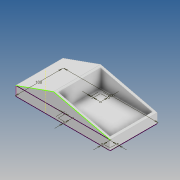
# Autodesk Inventor part: Cybertruck 1
Saved by Autodesk Inventor 2020 (Build 240168000, 168)
## iProperties
Created: 2019-11-26
Part Number: Cybertruck 1
Material: Generic
Document SubType Name: Modeling
Designer: Berkant
Density: 1 g/cm^3
Appearance: Default
Author: Berkant
Autodesk Inventor part; units mm, degrees
ref_plane "YZ Plane" through (0, 0, 0) normal (1, 0, 0) x (0, 1, 0)
ref_plane "XZ Plane" through (0, 0, 0) normal (0, 1, 0) x (-1, 0, 0)
ref_plane "XY Plane" through (0, 0, 0) normal (0, 0, 1) x (1, 0, 0)
sketch "Sketch1" plane through (0, 0, 0) normal (0, 1, 0) x (-1, 0, 0)
  line L0 (0, 0) -> (200, 0)
  line L1 (200, 0) -> (200, -100)
  line L2 (200, -100) -> (0, -100)
  line L3 (0, -100) -> (0, 0)
  dimension "d0" = 200
  dimension "d1" = 100
  constraints: 8 end point, 2 parallel, 1 horizontal, 1 perpendicular
  measures "d0" distance of L1.end L2.end
  measures "d1" distance of L0.end L1.end
extrude "Extrusion1" add sketch "Sketch1" along normal blind 20
sketch "Sketch2" plane through (-200, 0, 0) normal (0, 0, 1) x (1, 0, 0)
  line L0 (0, 0) -> (0, 20) projected
  line L1 (0, 0) -> (32, 0)
  line L2 (32, 0) -> (64, 0)
  line L3 (200, 0) -> (0, 0) projected
  line L4 (64, 0) -> (96, 0)
  line L5 (96, 0) -> (128, 0)
  line L6 (128, 0) -> (200, 0)
  line L7 (64, 0) -> (64, 80.3945) construction
  line L8 (200, 20) -> (0, 20) projected
  line L9 (0, 20) -> (200, 20)
  line L10 (0, 20) -> (200, 20) projected
  line L11 (0, 20) -> (200, 20)
  line L12 (0, 20) -> (80, 48.5382)
  line L13 (80, 48.5382) -> (200, 20)
  constraints: 20 end point, 3 collinear, 3 point on line, 1 horizontal, 1 vertical
extrude "Extrusion2" add sketch "Sketch2" against normal blind 100
sketch "Sketch4" plane through (0, 0, 0) normal (0, -1, 0) x (1, 0, 0)
  line L0 (0, 0) -> (-5, 0)
  line L1 (-5, 0) -> (-5, -5)
  line L2 (-5, -5) -> (0, -5)
  line L3 (0, -5) -> (0, 0)
  line L4 (-120, 0) -> (-120, -100) projected
  line L5 (-120, 0) -> (-115, 0)
  line L6 (-115, 0) -> (-115, -5)
  line L7 (-115, -5) -> (-120, -5)
  line L8 (-120, -5) -> (-120, 0)
  line L9 (-120, -100) -> (-115, -100)
  line L10 (-115, -100) -> (-115, -95)
  line L11 (-115, -95) -> (-120, -95)
  line L12 (-120, -95) -> (-120, -100)
  line L13 (-115, -5) -> (-5, -5)
  line L14 (-5, -5) -> (-5, -95)
  line L15 (-5, -95) -> (-115, -95)
  line L16 (-115, -95) -> (-115, -5)
  dimension "d23" = 5
  dimension "d24" = 5
  dimension "d25" = 5
  dimension "d26" = 5
  dimension "d27" = 5
  dimension "d28" = 5
  constraints: 32 end point, 8 parallel, 4 horizontal, 4 perpendicular
  measures "d23" distance of L2.end L1.end
  measures "d24" distance of L1.end L0.end
  measures "d25" distance of L6.end L7.end
  measures "d26" distance of L5.end L6.end
  measures "d27" distance of L11.end L10.end
  measures "d28" distance of L10.end L9.end
extrude "Extrusion3" cut sketch "Sketch4" against normal blind 68.75 contours L14 L15 L16 L13
extrude "Extrusion4" add sketch "Sketch4" against normal blind 10 contours L14 L15 L16 L13
body "Solid1"
